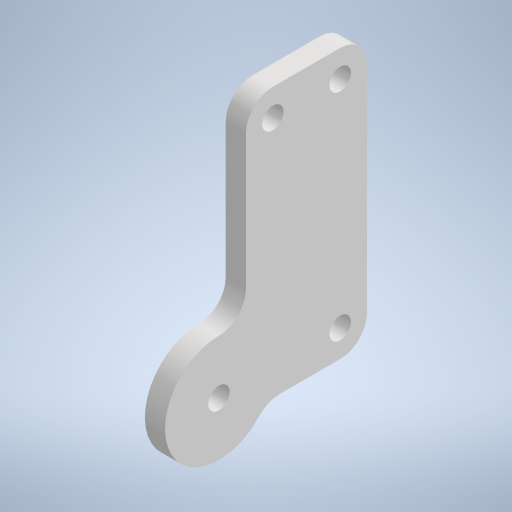
# Autodesk Inventor part: chest_cover_side_joint
Saved by Autodesk Inventor 2024.1 (Build 281209000, 209)
## iProperties
Created: 2024-02-15
Part Number: chest_cover_side_joint
Material: 一般
Document SubType Name: Modeling
Designer: hibik
Density: 1 g/cm^3
Appearance: 既定
Author: hibik
Autodesk Inventor part; units mm, degrees
ref_plane "YZ Plane" through (0, 0, 0) normal (1, 0, 0) x (0, 1, 0)
ref_plane "XZ Plane" through (0, 0, 0) normal (0, 1, 0) x (-1, 0, 0)
ref_plane "XY Plane" through (0, 0, 0) normal (0, 0, 1) x (1, 0, 0)
sketch "スケッチ1" plane through (0, 0, 0) normal (1, 0, 0) x (0, 1, 0)
  line L0 (20, 0) -> (0, 0)
  line L1 (0, 0) -> (0, -9)
  line L2 (0, -9) -> (20, -9)
  line L3 (20, -9) -> (20, 0)
  circle A0 centre (2, 2) radius 2
  circle A1 centre (2, 2) radius 0.8
  line L4 (4, 4) -> (0, 4)
  line L5 (0, 4) -> (0, 0)
  line L6 (0, 0) -> (4, 0)
  line L7 (4, 0) -> (4, 4)
  circle A2 centre (2, 2) radius 4
  point P0 (4, 2)
  point P1 (0, 2)
  point P2 (5.4641, 0)
  point P3 (0, -1.4641)
  dimension "d0" = 4
  dimension "d1" = 1.6
  dimension "d2" = 9
  dimension "d3" = 20
  dimension "d12" = 8
  constraints: 16 end point, 4 parallel, 4 tangent, 3 centre point, 3 coincident, 2 collinear, 2 horizontal, 2 perpendicular
  measures "d0" diameter of A0
  measures "d1" diameter of A1
  measures "d2" distance of L2.end L0.start
  measures "d3" distance of L1.end L2.end
  measures "d12" diameter of A2
extrude "押し出し1" add sketch "スケッチ1" along normal blind 1.5
fillet "フィレット1" radius 2 5 edges at (0.75, 20, 0) (0.75, 20, -9) (0.75, 0, -9) (0.75, 0, -1.4641) (0.75, 5.4641, 0)
sketch "スケッチ2" plane through (1.5, 0, 0) normal (1, 0, 0) x (0, 0, -1)
  circle A0 centre (2, 18) radius 0.8
  circle A1 centre (7, 18) radius 0.8
  circle A2 centre (7, 2) radius 0.8
  arc A3 (9, 18) -> (7, 20) centre (7, 18) ccw projected
  arc A4 (2, 20) -> (0, 18) centre (2, 18) ccw projected
  arc A5 (7, 0) -> (9, 2) centre (7, 2) ccw projected
  point P0 (0, 0)
  dimension "d6" = 1.6
  dimension "d7" = 1.6
  dimension "d8" = 1.6
  constraints: 3 centre point, 3 concentric
  measures "d6" diameter of A0
  measures "d7" diameter of A1
  measures "d8" diameter of A2
extrude "押し出し2" cut sketch "スケッチ2" against normal through all
